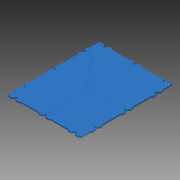
# Autodesk Inventor part: Bottom Panel
Saved by Autodesk Inventor 2014 (Build 180170000, 170)
## iProperties
Created: 2013-09-27
Part Number: Bottom Panel
Material: Generic
Document SubType Name: Modeling
Designer: TechShop Member
Density: 1 g/cm^3
Appearance: Default
Author: TechShop Member
Autodesk Inventor part; units mm, degrees
ref_plane "YZ Plane" through (0, 0, 0) normal (1, 0, 0) x (0, 1, 0)
ref_plane "XZ Plane" through (0, 0, 0) normal (0, 1, 0) x (-1, 0, 0)
ref_plane "XY Plane" through (0, 0, 0) normal (0, 0, 1) x (1, 0, 0)
sketch "Block1" plane through (0, 0, 0) normal (0, 0, 1) x (1, 0, 0)
  line L0 (-103.629, -133.35) -> (-103.629, -136.35)
  line L1 (-103.629, -136.35) -> (-93.479, -136.35)
  line L2 (-93.479, -136.35) -> (-93.479, -133.35)
  line L3 (-88.979, -133.35) -> (-88.979, -131.35)
  line L4 (-88.979, -131.35) -> (-90.229, -131.35)
  line L5 (-90.229, -131.35) -> (-90.229, -128.95)
  line L6 (-90.229, -128.95) -> (-88.979, -128.95)
  line L7 (-88.979, -128.95) -> (-88.979, -126.95)
  line L8 (-88.979, -126.95) -> (-85.979, -126.95)
  line L9 (-85.979, -126.95) -> (-85.979, -128.95)
  line L10 (-85.979, -128.95) -> (-84.729, -128.95)
  line L11 (-84.729, -128.95) -> (-84.729, -131.35)
  line L12 (-84.729, -131.35) -> (-85.979, -131.35)
  line L13 (-85.979, -131.35) -> (-85.979, -133.35)
  line L14 (-88.979, -133.35) -> (-93.479, -133.35)
  line L15 (-81.479, -133.35) -> (-81.479, -136.35)
  line L16 (-81.479, -136.35) -> (-71.329, -136.35)
  line L17 (-71.329, -136.35) -> (-71.329, -133.35)
  line L18 (-81.479, -133.35) -> (-85.979, -133.35)
  point P0 (-87.7527, -132.0076)
  dimension "d107" = 3
  dimension "d108" = 10.15
  measures "d107" distance of L0.start L0.end
  measures "d108" distance of L0.end L1.end
sketch "Sketch1" plane through (0, 0, 0) normal (0, 1, 0) x (-1, 0, 0)
  line L0 (107.5, -133.35) -> (103.629, -133.35)
  line L1 (-107.5, -133.3478) -> (-107.5, -105.0478)
  line L2 (-107.5, 133.3522) -> (-103.5759, 133.3522)
  line L3 (107.5, 133.3522) -> (107.5, 105.05)
  line L4 (-155.228, -77.2893) -> (-155.228, -80.2893)
  line L5 (-145.1277, -77.2893) -> (-145.1277, -80.2893)
  line L6 (-155.228, -77.2893) -> (-145.1277, -77.2893)
  line L7 (-133.1284, -77.2893) -> (-133.1284, -80.2893)
  line L8 (-123.0281, -77.2893) -> (-123.0281, -80.2893)
  line L9 (-133.1284, -77.2893) -> (-123.0281, -77.2893)
  line L10 (-140.628, -80.2893) -> (-140.628, -82.2891)
  line L11 (-140.628, -82.2891) -> (-141.8781, -82.2891)
  line L12 (-141.8781, -82.2891) -> (-141.8781, -84.689)
  line L13 (-140.628, -84.689) -> (-141.8781, -84.689)
  line L14 (-140.628, -84.689) -> (-140.628, -86.6889)
  line L15 (-140.6692, -86.6889) -> (-137.6692, -86.6889)
  line L16 (-137.6692, -84.689) -> (-137.6692, -86.6889)
  line L17 (-136.4193, -84.689) -> (-137.6692, -84.689)
  line L18 (-136.4193, -82.2891) -> (-136.4193, -84.689)
  line L19 (-136.3782, -82.2891) -> (-137.6281, -82.2891)
  line L20 (-137.6281, -80.2893) -> (-137.6281, -82.2891)
  line L21 (-140.628, -80.2893) -> (-145.1277, -80.2893)
  line L22 (-137.6281, -80.2893) -> (-133.1284, -80.2893)
  line L23 (103.629, 133.3522) -> (103.629, 136.35)
  line L24 (103.629, 136.35) -> (93.479, 136.35)
  line L25 (93.479, 136.35) -> (93.479, 133.35)
  line L26 (103.629, 133.3522) -> (107.5, 133.3522)
  line L27 (93.479, 133.35) -> (88.979, 133.35)
  line L28 (88.979, 133.35) -> (88.979, 131.35)
  line L29 (88.979, 131.35) -> (90.229, 131.35)
  line L30 (90.229, 131.35) -> (90.229, 128.95)
  line L31 (90.229, 128.95) -> (88.7898, 128.95)
  line L32 (88.7898, 128.95) -> (88.7898, 126.95)
  line L33 (88.7898, 126.95) -> (85.7898, 126.95)
  line L34 (85.7898, 126.95) -> (85.7898, 128.95)
  line L35 (85.7898, 128.95) -> (84.5398, 128.95)
  line L36 (84.5398, 128.95) -> (84.5398, 131.35)
  line L37 (84.5398, 131.35) -> (86.0328, 131.35)
  line L38 (86.0328, 131.35) -> (86.0328, 133.35)
  line L39 (88.979, 133.35) -> (93.479, 133.35)
  line L40 (81.5328, 133.35) -> (81.5328, 136.35)
  line L41 (81.5328, 136.35) -> (71.3828, 136.35)
  line L42 (71.3828, 136.35) -> (71.3828, 133.35)
  line L43 (81.5328, 133.35) -> (86.0328, 133.35)
  line L44 (16.1875, 133.35) -> (16.1875, 136.35)
  line L45 (16.1875, 136.35) -> (6.0375, 136.35)
  line L46 (6.0375, 136.35) -> (6.0375, 133.35)
  line L47 (1.5375, 133.35) -> (1.5375, 131.35)
  line L48 (1.5375, 131.35) -> (2.7875, 131.35)
  line L49 (2.7875, 131.35) -> (2.7875, 128.95)
  line L50 (2.7875, 128.95) -> (1.5375, 128.95)
  line L51 (1.5375, 128.95) -> (1.5375, 126.95)
  line L52 (1.5375, 126.95) -> (-1.4625, 126.95)
  line L53 (-1.4625, 126.95) -> (-1.4625, 128.95)
  line L54 (-1.4625, 128.95) -> (-2.7125, 128.95)
  line L55 (-2.7125, 128.95) -> (-2.7125, 131.35)
  line L56 (-2.7125, 131.35) -> (-1.4625, 131.35)
  line L57 (-1.4625, 131.35) -> (-1.4625, 133.35)
  line L58 (-5.9625, 133.35) -> (-5.9625, 136.35)
  line L59 (-5.9625, 136.35) -> (-16.1125, 136.35)
  line L60 (-16.1125, 136.35) -> (-16.1125, 133.35)
  line L61 (16.1875, 133.35) -> (71.3828, 133.35)
  line L62 (1.5375, 133.35) -> (6.0375, 133.35)
  line L63 (-5.9625, 133.35) -> (-1.4625, 133.35)
  line L64 (-103.5759, 133.3522) -> (-103.5752, 136.3522)
  line L65 (-103.5752, 136.3522) -> (-93.4252, 136.3497)
  line L66 (-93.4252, 136.3497) -> (-93.4252, 133.35)
  line L67 (-88.9252, 133.35) -> (-88.9252, 131.35)
  line L68 (-88.9252, 131.35) -> (-90.1752, 131.35)
  line L69 (-90.1752, 131.35) -> (-90.1752, 128.95)
  line L70 (-90.1752, 128.95) -> (-88.9252, 128.95)
  line L71 (-88.9252, 128.95) -> (-88.9252, 126.95)
  line L72 (-88.9252, 126.95) -> (-85.9252, 126.95)
  line L73 (-85.9252, 126.95) -> (-85.9252, 128.95)
  line L74 (-85.9252, 128.95) -> (-84.6752, 128.95)
  line L75 (-84.6752, 128.95) -> (-84.6752, 131.35)
  line L76 (-84.6752, 131.35) -> (-85.9252, 131.35)
  line L77 (-85.9252, 131.35) -> (-85.9252, 133.35)
  line L78 (-81.4252, 133.35) -> (-81.4252, 136.35)
  line L79 (-81.4252, 136.35) -> (-71.2752, 136.35)
  line L80 (-71.2752, 136.35) -> (-71.2752, 133.35)
  line L81 (-71.2752, 133.35) -> (-16.1125, 133.35)
  line L82 (-85.9252, 133.35) -> (-81.4252, 133.35)
  line L83 (-93.4252, 133.35) -> (-88.9252, 133.35)
  line L84 (103.629, -133.35) -> (103.629, -136.35)
  line L85 (103.629, -136.35) -> (93.479, -136.35)
  line L86 (93.479, -136.35) -> (93.479, -133.35)
  line L87 (93.479, -133.35) -> (88.7523, -133.35)
  line L88 (88.7523, -133.35) -> (88.7523, -131.35)
  line L89 (88.7523, -131.35) -> (90.0023, -131.35)
  line L90 (90.0023, -131.35) -> (90.0023, -128.95)
  line L91 (90.0023, -128.95) -> (88.7523, -128.95)
  line L92 (88.7523, -128.95) -> (88.7523, -126.95)
  line L93 (88.7523, -126.95) -> (85.7523, -126.95)
  line L94 (85.7523, -126.95) -> (85.7523, -128.95)
  line L95 (85.7523, -128.95) -> (84.5023, -128.95)
  line L96 (84.5023, -128.95) -> (84.5023, -131.35)
  line L97 (84.5023, -131.35) -> (85.7686, -131.35)
  line L98 (85.7686, -131.35) -> (85.7686, -133.35)
  line L99 (85.7686, -133.35) -> (81.2686, -133.35)
  line L100 (81.2686, -133.35) -> (81.2686, -136.35)
  line L101 (81.2686, -136.35) -> (71.1186, -136.35)
  line L102 (71.1186, -136.35) -> (71.1186, -133.35)
  line L103 (71.1186, -133.35) -> (16.1663, -133.35)
  line L104 (16.1663, -133.35) -> (16.1663, -136.35)
  line L105 (16.1663, -136.35) -> (6.0163, -136.35)
  line L106 (6.0163, -136.35) -> (6.0163, -133.35)
  line L107 (6.0163, -133.35) -> (1.5163, -133.35)
  line L108 (1.5163, -133.35) -> (1.5163, -131.35)
  line L109 (1.5163, -131.35) -> (2.7663, -131.35)
  line L110 (2.7663, -131.35) -> (2.7663, -128.95)
  line L111 (2.7663, -128.95) -> (1.5163, -128.95)
  line L112 (1.5163, -128.95) -> (1.5163, -126.95)
  line L113 (1.5163, -126.95) -> (-1.5163, -126.95)
  line L114 (-1.5163, -126.95) -> (-1.5163, -128.9478)
  line L115 (-1.5163, -128.9478) -> (-2.7663, -128.9478)
  line L116 (-2.7663, -128.9478) -> (-2.7663, -131.3478)
  line L117 (-2.7663, -131.3478) -> (-1.5163, -131.3478)
  line L118 (-1.5163, -131.3478) -> (-1.5163, -133.3478)
  line L119 (-1.5163, -133.3478) -> (-6.0163, -133.3478)
  line L120 (-6.0163, -133.3478) -> (-6.0163, -136.3478)
  line L121 (-6.0163, -136.3478) -> (-16.1663, -136.3478)
  line L122 (-16.1663, -136.3478) -> (-16.1663, -133.3478)
  line L123 (-16.1663, -133.3478) -> (-71.3127, -133.3478)
  line L124 (-103.6127, -133.3478) -> (-107.5, -133.3478)
  line L125 (-107.5, -72.75) -> (-107.5, -16.15)
  line L126 (-71.3127, -133.3478) -> (-71.3127, -136.35)
  line L127 (-71.3127, -136.35) -> (-81.4627, -136.35)
  line L128 (-81.4627, -136.35) -> (-81.4627, -133.35)
  line L129 (-81.4627, -133.35) -> (-85.9627, -133.35)
  line L130 (-85.9627, -133.35) -> (-85.9627, -131.35)
  line L131 (-85.9627, -131.35) -> (-84.7127, -131.35)
  line L132 (-84.7127, -131.35) -> (-84.7127, -128.95)
  line L133 (-84.7127, -128.95) -> (-85.9627, -128.95)
  line L134 (-85.9627, -128.95) -> (-85.9627, -126.95)
  line L135 (-85.9627, -126.95) -> (-88.9627, -126.95)
  line L136 (-88.9627, -126.95) -> (-88.9627, -128.9478)
  line L137 (-88.9627, -128.9478) -> (-90.2127, -128.9478)
  line L138 (-90.2127, -128.9478) -> (-90.2127, -131.3478)
  line L139 (-90.2127, -131.3478) -> (-88.9627, -131.3478)
  line L140 (-88.9627, -131.3478) -> (-88.9627, -133.3478)
  line L141 (-88.9627, -133.3478) -> (-93.4627, -133.3478)
  line L142 (-93.4627, -133.3478) -> (-93.4627, -136.3478)
  line L143 (-93.4627, -136.3478) -> (-103.6127, -136.3478)
  line L144 (-103.6127, -136.3478) -> (-103.6127, -133.3478)
  line L145 (-107.5, -105.0478) -> (-110.5, -105.0478)
  line L146 (-110.5, -105.0478) -> (-110.5, -94.8978)
  line L147 (-110.5, -94.8978) -> (-107.5, -94.8978)
  line L148 (-107.5, -94.8978) -> (-107.5, -90.3978)
  line L149 (-107.5, -90.3978) -> (-105.5, -90.3978)
  line L150 (-105.5, -90.3978) -> (-105.5, -91.6478)
  line L151 (-105.5, -91.6478) -> (-103.1, -91.6478)
  line L152 (-103.1, -91.6478) -> (-103.1, -90.3978)
  line L153 (-103.1, -90.3978) -> (-101.1, -90.3978)
  line L154 (-101.1, -90.3978) -> (-101.1, -87.3978)
  line L155 (-101.1, -87.3978) -> (-103.1, -87.3978)
  line L156 (-103.1, -87.3978) -> (-103.1, -86.1478)
  line L157 (-103.1, -86.1478) -> (-105.5, -86.1478)
  line L158 (-105.5, -86.1478) -> (-105.5, -87.4)
  line L159 (-105.5, -87.4) -> (-107.5, -87.4)
  line L160 (-107.5, -87.4) -> (-107.5, -82.9)
  line L161 (-107.5, -82.9) -> (-110.5, -82.9)
  line L162 (-110.5, -82.9) -> (-110.5, -72.75)
  line L163 (-110.5, -72.75) -> (-107.5, -72.75)
  line L164 (-107.5, 16.15) -> (-107.5, 72.75)
  line L165 (-107.5, -16.15) -> (-110.5, -16.15)
  line L166 (-110.5, -16.15) -> (-110.5, -6)
  line L167 (-110.5, -6) -> (-107.5, -6)
  line L168 (-107.5, -6) -> (-107.5, -1.5)
  line L169 (-107.5, -1.5) -> (-105.5, -1.5)
  line L170 (-105.5, -1.5) -> (-105.5, -2.75)
  line L171 (-105.5, -2.75) -> (-103.1, -2.75)
  line L172 (-103.1, -2.75) -> (-103.1, -1.5)
  line L173 (-103.1, -1.5) -> (-101.1, -1.5)
  line L174 (-101.1, -1.5) -> (-101.1, 1.5)
  line L175 (-101.1, 1.5) -> (-103.1, 1.5)
  line L176 (-103.1, 1.5) -> (-103.1, 2.75)
  line L177 (-103.1, 2.75) -> (-105.5, 2.75)
  line L178 (-105.5, 2.75) -> (-105.5, 1.5)
  line L179 (-105.5, 1.5) -> (-107.5, 1.5)
  line L180 (-107.5, 1.5) -> (-107.5, 6)
  line L181 (-107.5, 6) -> (-110.5, 6)
  line L182 (-110.5, 6) -> (-110.5, 16.15)
  line L183 (-110.5, 16.15) -> (-107.5, 16.15)
  line L184 (-105.538, 133.3522) -> (-105.538, 105.0522)
  line L185 (-107.5, 105.05) -> (-107.5, 133.3522)
  line L186 (-107.5, 105.05) -> (-110.5, 105.05)
  line L187 (-110.5, 105.05) -> (-110.5, 94.9)
  line L188 (-110.5, 94.9) -> (-107.5, 94.9)
  line L189 (-107.5, 94.9) -> (-107.5, 90.4)
  line L190 (-107.5, 90.4) -> (-105.5, 90.4)
  line L191 (-105.5, 90.4) -> (-105.5, 91.65)
  line L192 (-105.5, 91.65) -> (-103.1, 91.65)
  line L193 (-103.1, 91.65) -> (-103.1, 90.4)
  line L194 (-103.1, 90.4) -> (-101.1, 90.4)
  line L195 (-101.1, 90.4) -> (-101.1, 87.4)
  line L196 (-101.1, 87.4) -> (-103.1, 87.4)
  line L197 (-103.1, 87.4) -> (-103.1, 86.15)
  line L198 (-103.1, 86.15) -> (-105.5, 86.15)
  line L199 (-105.5, 86.15) -> (-105.5, 87.4)
  line L200 (-105.5, 87.4) -> (-107.5, 87.4)
  line L201 (-107.5, 87.4) -> (-107.5, 82.9)
  line L202 (-107.5, 82.9) -> (-110.5, 82.9)
  line L203 (-110.5, 82.9) -> (-110.5, 72.75)
  line L204 (-110.5, 72.75) -> (-107.5, 72.75)
  line L205 (107.5, -105.05) -> (107.5, -133.35)
  line L206 (107.5, -105.05) -> (110.5, -105.05)
  line L207 (110.5, -105.05) -> (110.5, -94.9)
  line L208 (110.5, -94.9) -> (107.5, -94.9)
  line L209 (107.5, -94.9) -> (107.5, -90.4)
  line L210 (107.5, -90.4) -> (105.5, -90.4)
  line L211 (105.5, -90.4) -> (105.5, -91.65)
  line L212 (105.5, -91.65) -> (103.1, -91.65)
  line L213 (103.1, -91.65) -> (103.1, -90.4)
  line L214 (103.1, -90.4) -> (101.1, -90.4)
  line L215 (101.1, -90.4) -> (101.1, -87.4)
  line L216 (101.1, -87.4) -> (103.1, -87.4)
  line L217 (103.1, -87.4) -> (103.1, -86.15)
  line L218 (103.1, -86.15) -> (105.5, -86.15)
  line L219 (105.5, -86.15) -> (105.5, -87.4)
  line L220 (105.5, -87.4) -> (107.5, -87.4)
  line L221 (107.5, -87.4) -> (107.5, -82.9)
  line L222 (107.5, -82.9) -> (110.5, -82.9)
  line L223 (110.5, -82.9) -> (110.5, -72.75)
  line L224 (110.5, -72.75) -> (107.5, -72.75)
  line L225 (107.5, 72.55) -> (107.5, 16.15)
  line L226 (107.5, 105.05) -> (110.5, 105.05)
  line L227 (110.5, 105.05) -> (110.5, 94.9)
  line L228 (110.5, 94.9) -> (107.5, 94.9)
  line L229 (107.5, 94.9) -> (107.5, 90.4)
  line L230 (107.5, 90.4) -> (105.5, 90.4)
  line L231 (105.5, 90.4) -> (105.5, 91.65)
  line L232 (105.5, 91.65) -> (103.1, 91.65)
  line L233 (103.1, 91.65) -> (103.1, 90.4)
  line L234 (103.1, 90.4) -> (101.1, 90.4)
  line L235 (101.1, 90.4) -> (101.1, 87.4)
  line L236 (101.1, 87.4) -> (103.1, 87.4)
  line L237 (103.1, 87.4) -> (103.1, 86.15)
  line L238 (103.1, 86.15) -> (105.5, 86.15)
  line L239 (105.5, 86.15) -> (105.5, 87.4)
  line L240 (105.5, 87.4) -> (107.5, 87.4)
  line L241 (107.5, 87.4) -> (107.5, 82.9)
  line L242 (107.5, 82.9) -> (110.5, 82.9)
  line L243 (110.5, 82.9) -> (110.5, 72.55)
  line L244 (110.5, 72.55) -> (107.5, 72.55)
  line L245 (107.5, -16.15) -> (107.5, -72.75)
  line L246 (107.5, 16.15) -> (110.5, 16.15)
  line L247 (110.5, 16.15) -> (110.5, 6)
  line L248 (110.5, 6) -> (107.5, 6)
  line L249 (107.5, 6) -> (107.5, 1.5)
  line L250 (107.5, 1.5) -> (105.5, 1.5)
  line L251 (105.5, 1.5) -> (105.5, 2.75)
  line L252 (105.5, 2.75) -> (103.1, 2.75)
  line L253 (103.1, 2.75) -> (103.1, 1.5)
  line L254 (103.1, 1.5) -> (101.1, 1.5)
  line L255 (101.1, 1.5) -> (101.1, -1.5)
  line L256 (101.1, -1.5) -> (103.1, -1.5)
  line L257 (103.1, -1.5) -> (103.1, -2.75)
  line L258 (103.1, -2.75) -> (105.5, -2.75)
  line L259 (105.5, -2.75) -> (105.5, -1.5)
  line L260 (105.5, -1.5) -> (107.5, -1.5)
  line L261 (107.5, -1.5) -> (107.5, -6)
  line L262 (107.5, -6) -> (110.5, -6)
  line L263 (110.5, -6) -> (110.5, -16.15)
  line L264 (110.5, -16.15) -> (107.5, -16.15)
  point P0 (0, 0)
  point P1 (-139.1692, -82.8816)
  point P2 (-107.5, 122.7286)
  point P3 (-101.1, -88.8978)
  point P4 (-87.4627, -126.95)
  point P5 (0, -126.95)
  point P6 (87.2523, -126.95)
  point P7 (0.0375, 126.95)
  point P8 (-87.4252, 126.95)
  point P9 (87.2898, 126.95)
  dimension "d0" = 215
  dimension "d1" = 266.7
  dimension "d2" = 133.35
  dimension "d3" = 107.5
  dimension "d35" = 1.2499
  dimension "d36" = 1.2501
  dimension "d37" = 16.1411
  dimension "d40" = 3
  dimension "d41" = 10.1003
  dimension "d42" = 10.1003
  dimension "d43" = 3
  dimension "d45" = 10.15
  dimension "d46" = 4.4996
  dimension "d47" = 1.9999
  dimension "d48" = 2.3998
  dimension "d49" = 1.9999
  dimension "d50" = 3
  dimension "d51" = 4.5
  dimension "d53" = 1.25
  dimension "d54" = 2.4
  dimension "d55" = 2
  dimension "d56" = 3
  dimension "d57" = 1.25
  dimension "d58" = 2
  dimension "d59" = 4.4996
  dimension "d60" = 4.5
  dimension "d61" = 3
  dimension "d62" = 10.15
  dimension "d63" = 3
  dimension "d64" = 10.15
  dimension "d65" = 4.5
  dimension "d66" = 2
  dimension "d67" = 1.25
  dimension "d68" = 2.4
  dimension "d69" = 1.25
  dimension "d70" = 2
  dimension "d71" = 3
  dimension "d72" = 1.25
  dimension "d73" = 4.5
  dimension "d74" = 10.15
  dimension "d75" = 3.871
  dimension "d77" = 3
  dimension "d78" = 10.15
  dimension "d79" = 4.5
  dimension "d80" = 2
  dimension "d81" = 1.25
  dimension "d82" = 2.4
  dimension "d83" = 1.25
  dimension "d84" = 2
  dimension "d85" = 3
  dimension "d86" = 1.25
  dimension "d87" = 4.5
  dimension "d88" = 10.15
  dimension "d90" = 3
  dimension "d91" = 10.15
  dimension "d92" = 2
  dimension "d93" = 1.25
  dimension "d94" = 2.4
  dimension "d95" = 2
  dimension "d96" = 3
  dimension "d97" = 1.25
  dimension "d99" = 3
  dimension "d100" = 10.15
  dimension "d101" = 3
  constraints: 530 end point, 307 parallel, 295 perpendicular, 9 point on line, 8 horizontal, 7 midpoint, 4 collinear
  measures "d0" distance of L2.start L3.start
  measures "d1" distance of L1.start L2.start
  measures "d2" distance from line of L0 point (0, 0)
  measures "d3" distance from line of L3 point (0, 0)
  measures "d35" distance of L17.start L17.end
  measures "d36" distance of L13.start L13.end
  measures "d37" horizontal distance of point (-139.169, -82.882) L8.end
  measures "d40" distance of L8.start L8.end
  measures "d41" distance of L9.start L9.end
  measures "d42" distance of L6.start L6.end
  measures "d43" distance of L7.start L7.end
  measures "d45" distance of L23.end L24.end
  measures "d46" distance of L22.start L22.end
  measures "d47" distance of L20.start L20.end
  measures "d48" distance of L18.start L18.end
  measures "d49" distance of L16.start L16.end
  measures "d50" distance of L15.start L15.end
  measures "d51" distance of L25.end L27.end
  measures "d53" distance of L28.end L29.end
  measures "d54" distance of L29.end L30.end
  measures "d55" distance of L31.end L32.end
  measures "d56" distance of L32.end L33.end
  measures "d57" distance of L34.end L35.end
  measures "d58" distance of L27.end L28.end
  measures "d59" distance of L21.start L21.end
  measures "d60" distance of L38.end L40.start
  measures "d61" distance of L40.start L40.end
  measures "d62" distance of L40.end L41.end
  measures "d63" distance of L44.start L44.end
  measures "d64" distance of L44.end L45.end
  measures "d65" distance of L46.end L47.start
  measures "d66" distance of L47.start L47.end
  measures "d67" distance of L47.end L48.end
  measures "d68" distance of L48.end L49.end
  measures "d69" distance of L49.end L50.end
  measures "d70" distance of L50.end L51.end
  measures "d71" distance of L51.end L52.end
  measures "d72" distance of L53.end L54.end
  measures "d73" distance of L57.end L58.start
  measures "d74" distance of L58.end L59.end
  measures "d75" distance of L23.start L3.start
  measures "d77" distance of L2.end L64.end
  measures "d78" distance of L64.end L65.end
  measures "d79" distance of L66.end L67.start
  measures "d80" distance of L67.start L67.end
  measures "d81" distance of L67.end L68.end
  measures "d82" distance of L68.end L69.end
  measures "d83" distance of L69.end L70.end
  measures "d84" distance of L70.end L71.end
  measures "d85" distance of L71.end L72.end
  measures "d86" distance of L73.end L74.end
  measures "d87" distance of L77.end L78.start
  measures "d88" distance of L78.end L79.end
  measures "d90" distance of L0.end L84.end
  measures "d91" distance of L84.end L85.end
  measures "d92" distance of L87.end L88.end
  measures "d93" distance of L88.end L89.end
  measures "d94" distance of L89.end L90.end
  measures "d95" distance of L91.end L92.end
  measures "d96" distance of L92.end L93.end
  measures "d97" distance of L94.end L95.end
  measures "d99" distance of L99.end L100.end
  measures "d100" distance of L100.end L101.end
  measures "d101" distance of L103.end L104.end
extrude "Extrusion2" add sketch "Sketch1" along normal blind 3
equation "\"d2\" = 0.5 * d1"
equation "\"d3\" = 0.5 * d0"
body "Solid2"
